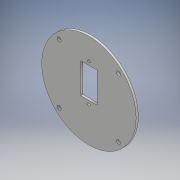
# Autodesk Inventor part: podstawa
Saved by Autodesk Inventor 2017.3 (Build 213256000, 256)
## iProperties
Created: 2019-03-17
Part Number: podstawa
Material: Ogólny
Document SubType Name: Modeling
Designer: legox
Density: 1 g/cm^3
Appearance: Domyślna
Author: legox
Autodesk Inventor part; units mm, degrees
ref_plane "YZ Plane" through (0, 0, 0) normal (1, 0, 0) x (0, 1, 0)
ref_plane "XZ Plane" through (0, 0, 0) normal (0, 1, 0) x (-1, 0, 0)
ref_plane "XY Plane" through (0, 0, 0) normal (0, 0, 1) x (1, 0, 0)
sketch "Szkic1" plane through (0, 0, 0) normal (0, 1, 0) x (-1, 0, 0)
  circle A0 centre (0, 0) radius 35
  line L0 (-6, -6.25) -> (6, -6.25)
  line L1 (6, -6.25) -> (6, 16.25)
  line L2 (6, 16.25) -> (-6, 16.25)
  line L3 (-6, 16.25) -> (-6, -6.25)
  circle A1 centre (0, 18.85) radius 1
  circle A2 centre (-22, -22) radius 1.5
  circle A3 centre (22, -22) radius 1.5
  circle A4 centre (22, 22) radius 1.5
  circle A5 centre (-22, 22) radius 1.5
  circle A6 centre (0, -8.85) radius 1
  dimension "d0" = 70
  dimension "d1" = 12
  dimension "d2" = 22.5
  dimension "d3" = 2
  dimension "d4" = 2.6
  dimension "d7" = 3
  dimension "d10" = 360
  dimension "d12" = 22
  dimension "d13" = 22
  dimension "d14" = 2
  dimension "d15" = 6
  dimension "d16" = 2.6
  dimension "d17" = 6
  dimension "d18" = 6.25
  constraints: 8 end point, 7 centre point, 2 parallel, 1 coincident, 1 horizontal, 1 perpendicular, 9 other
  measures "d0" diameter of A0
  measures "d1" distance of L2.end L1.end
  measures "d2" distance of L1.end L0.end
  measures "d3" diameter of A1
  measures "d4" distance from line of A1.centre L2
  measures "d7" diameter of A2
  measures "d12" horizontal distance of point (0, 0) A2.centre
  measures "d13" horizontal distance of point (0, 0) A2.centre
  measures "d14" diameter of A6
  measures "d15" distance from line of L3 A1.centre
  measures "d16" distance from line of L0 A6.centre
  measures "d17" distance from line of L3 A6.centre
  measures "d18" distance from line of point (0, 0) L0
extrude "Wyciągnięcie proste1" add sketch "Szkic1" along normal blind 1.6
equation "\"d15\" = 0.5 * d1"
equation "\"d17\" = 0.5 * d1"
